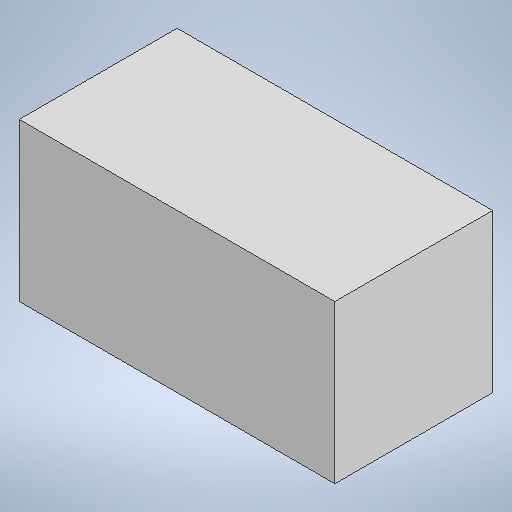
# Autodesk Inventor part: Nose_Camera
Saved by Autodesk Inventor 2027 (Build 310192000, 192)
## iProperties
Created: 2026-09-10
Part Number: Nose_Camera
Material: Generic
Document SubType Name: Modeling
Designer: IG2
Density: 1 g/cm^3
Appearance: Default
Author: IG2
Autodesk Inventor part; units mm, degrees
ref_plane "YZ Plane" through (0, 0, 0) normal (1, 0, 0) x (0, 1, 0)
ref_plane "XZ Plane" through (0, 0, 0) normal (0, 1, 0) x (-1, 0, 0)
ref_plane "XY Plane" through (0, 0, 0) normal (0, 0, 1) x (1, 0, 0)
sketch "Sketch1" plane through (0, 0, 0) normal (0, 0, 1) x (1, 0, 0)
  line L0 (-30, 17.1429) -> (30, 17.1429)
  line L1 (30, 17.1429) -> (30, -12.8571)
  line L2 (30, -12.8571) -> (-30, -12.8571)
  line L3 (-30, -12.8571) -> (-30, 17.1429)
  line L4 (0, 17.1429) -> (0, -12.8571)
  point P0 (0, 0)
  dimension "d1" = 60
  dimension "d2" = 30
  constraints: 10 end point, 2 midpoint, 2 parallel, 2 perpendicular, 1 horizontal
  measures "d1" distance between parallel lines of L1 L3
  measures "d2" distance between parallel lines of L2 L0
extrude "Extrusion1" add sketch "Sketch1" along normal mid plane 30
body "Solid1"
